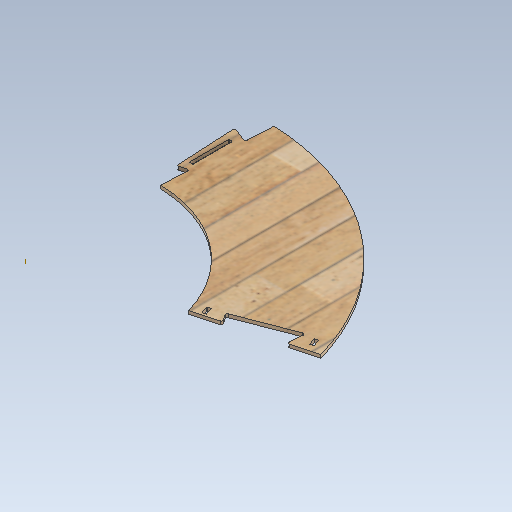
# Autodesk Inventor part: Ring C3
Saved by Autodesk Inventor 2020 (Build 240168000, 168)
## iProperties
Created: 2020-03-10
Part Number: Ring C3
Material: Wood (Maple)
Document SubType Name: Sheet Metal
Designer: Daniel Wikman
Density: 0.67 g/cm^3
Sheet Metal Rule: Default_mm
Appearance: Natural Maple - Glossy Dark Tint
Author: Daniel Wikman
Autodesk Inventor part; units mm, degrees
ref_plane "YZ Plane" through (0, 0, 0) normal (1, 0, 0) x (0, 1, 0)
ref_plane "XZ Plane" through (0, 0, 0) normal (0, 1, 0) x (-1, 0, 0)
ref_plane "XY Plane" through (0, 0, 0) normal (0, 0, 1) x (1, 0, 0)
sketch "Sketch1" plane through (0, 0, 0) normal (0, 1, 0) x (-1, 0, 0)
  circle A0 centre (0, 0) radius 425
  circle A1 centre (0, 0) radius 233.71
  dimension "d84" = 467.42
  dimension "d85" = 850
  constraints: 2 centre point, 1 coincident
  measures "d84" diameter of A1
  measures "d85" diameter of A0
extrude "Extrusion3" add sketch "Sketch1" along normal blind 6
sketch "Sketch2" plane through (0, 6, 0) normal (0, 1, 0) x (1, 0, 0)
  circle A0 centre (0, 0) radius 329.355 construction
  line L0 (3.25, 363.0217) -> (3.25, 295.6883)
  line L1 (-3.25, 295.6883) -> (-3.25, 363.0217)
  arc A1 (-3.25, 295.6883) -> (-1.9167, 294.355) centre (-1.9167, 295.6883) ccw
  arc A2 (1.9167, 294.355) -> (3.25, 295.6883) centre (1.9167, 295.6883) ccw
  arc A3 (-1.9167, 364.355) -> (-3.25, 363.0217) centre (-1.9167, 363.0217) ccw
  arc A4 (3.25, 363.0217) -> (1.9167, 364.355) centre (1.9167, 363.0217) ccw
  line L2 (-1.9167, 364.355) -> (1.9167, 364.355)
  line L3 (-1.9167, 294.355) -> (1.9167, 294.355)
  line L4 (0, 294.355) -> (0, 329.355) construction
  line L5 (0, 364.355) -> (0, 329.355) construction
  line L6 (0, 364.355) -> (0, 294.355) construction
  line L7 (175.0629, -238.5433) -> (171.9617, -240.7965)
  arc A5 (176.9253, -238.8383) -> (175.0629, -238.5433) centre (175.8467, -239.622) ccw
  arc A6 (171.9617, -240.7965) -> (171.6667, -242.6589) centre (172.7454, -241.8752) ccw
  line L8 (173.0175, -238.1382) -> (193.59, -266.4538) construction
  line L9 (211.2443, -297.1327) -> (171.6667, -242.6589)
  line L10 (176.9253, -238.8383) -> (216.5029, -293.3121)
  line L11 (214.1625, -294.7694) -> (173.0175, -238.1382) construction
  line L12 (214.1625, -294.7694) -> (193.59, -266.4538) construction
  arc A7 (211.2443, -297.1327) -> (213.1067, -297.4277) centre (212.323, -296.349) ccw
  line L13 (216.2079, -295.1745) -> (213.1067, -297.4277)
  arc A8 (216.2079, -295.1745) -> (216.5029, -293.3121) centre (215.4242, -294.0958) ccw
  line L14 (280.1548, 92.2019) -> (281.3393, 88.5562)
  arc A9 (281.0108, 93.882) -> (280.1548, 92.2019) centre (281.4229, 92.614) ccw
  arc A10 (281.3393, 88.5562) -> (283.0194, 87.7002) centre (282.6074, 88.9682) ccw
  line L15 (279.9482, 90.9607) -> (313.2352, 101.7763) construction
  line L16 (347.0573, 108.5073) -> (283.0194, 87.7002)
  line L17 (281.0108, 93.882) -> (345.0486, 114.6892)
  line L18 (346.5222, 112.5919) -> (279.9482, 90.9607) construction
  line L19 (346.5222, 112.5919) -> (313.2352, 101.7763) construction
  arc A11 (347.0573, 108.5073) -> (347.9133, 110.1874) centre (346.6452, 109.7754) ccw
  line L20 (346.7287, 113.8331) -> (347.9133, 110.1874)
  arc A12 (346.7287, 113.8331) -> (345.0486, 114.6892) centre (345.4607, 113.4211) ccw
  dimension "d86" = 658.71
  dimension "d21" = 6.5
  dimension "d24" = 2.6667
  dimension "d25" = 2.6667
  dimension "d32" = 1.3333
  dimension "d33" = 1.3333
  dimension "d162" = 70
  dimension "d163" = 294.355
  dimension "d165" = 3.25
  constraints: 42 end point, 24 point on circle, 12 centre point, 8 tangent, 2 midpoint, 1 coincident, 1 parallel, 1 vertical, 1 vertical alignment, 3 other
  measures "d21" distance between parallel lines of L0 L1
  measures "d24" diameter of A1
  measures "d25" diameter of A2
  measures "d32" radius of A3
  measures "d33" radius of A4
  measures "d162" distance between parallel lines of L3 L2
  measures "d163" distance from line of point (0, 0) L3
  measures "d165" distance between parallel lines of L5 L1
extrude "Extrusion4" cut sketch "Sketch2" against normal through all
sketch "Sketch3" plane through (0, 6, 0) normal (0, 1, 0) x (1, 0, 0)
  arc A0 (-131.3389, -404.1968) -> (131.3445, -404.195) centre (0, 0) ccw
  arc A1 (-77.7244, -128.3741) -> (77.7297, -128.3709) centre (0, 0) ccw
  line L0 (-122.1811, -173.696) -> (-161.3589, -227.6196)
  line L1 (-131.3389, -404.1968) -> (-77.7244, -128.3741)
  line L2 (0, 0) -> (0, -341.2918)
  line L3 (131.3445, -404.195) -> (77.7297, -128.3709)
  line L4 (210.5535, -295.3313) -> (171.3679, -241.3969) projected
  dimension "d52" = 25
  dimension "d87" = 150.07
  dimension "d88" = 425
  dimension "d89" = 25
  dimension "d90" = 11
  dimension "d91" = 11
  constraints: 8 end point, 4 point on circle, 2 centre point, 1 coincident
  measures "d52" angle of L0 L1
  measures "d87" radius of A1
  measures "d88" radius of A0
  measures "d89" angle of L4 L3
  measures "d90" angle of L3 L2
  measures "d91" angle of L1 L2
sketch "Sketch5" plane through (0, 6, 0) normal (0, 1, 0) x (1, 0, 0)
  line L0 (3.25, 363.0217) -> (3.25, 295.6883) projected
  line L1 (5.5862, 281.6788) -> (-6.155, 278.5328)
  line L2 (-11.2263, 385.43) -> (10.5847, 377.0575)
  line L3 (6.5657, 233.6709) -> (8.9394, 278.9635)
  line L4 (14.2034, 379.4075) -> (16.5771, 424.7001)
  arc A0 (10.5847, 377.0575) -> (14.2034, 379.4075) centre (11.5404, 379.5471) ccw
  arc A1 (8.9394, 278.9635) -> (5.5862, 281.6788) centre (6.2763, 279.103) ccw
  arc A2 (-11.2263, 385.43) -> (-14.8449, 382.8009) centre (-12.1819, 382.9405) ccw
  line L5 (-3.25, 295.6883) -> (-3.25, 363.0217) projected
  line L6 (-14.8449, 382.8009) -> (-9.5081, 280.969)
  arc A3 (-9.5081, 280.969) -> (-6.155, 278.5328) centre (-6.8451, 281.1086) ccw
  line L7 (-1.9167, 294.355) -> (1.9167, 294.355) projected
  line L8 (1.9167, 364.355) -> (-1.9167, 364.355) projected
  line L9 (16.5771, 424.7001) -> (16.5774, 424.7058)
  line L10 (6.5657, 233.6709) -> (6.5621, 233.6028)
  circle A4 centre (0, 0) radius 425
  circle A5 centre (0, 0) radius 233.71
  line L11 (-356.4489, 130.7516) -> (-398.7912, 147.0053)
  arc A6 (-355.3322, 126.5839) -> (-356.4489, 130.7516) centre (-357.4046, 128.2621) ccw
  line L12 (-370.0348, 108.4276) -> (-355.3322, 126.5839)
  arc A7 (-370.0348, 108.4276) -> (-368.6526, 104.1736) centre (-367.9624, 106.7494) ccw
  line L13 (-368.6526, 104.1736) -> (-270.1556, 77.7814)
  arc A8 (-270.1556, 77.7814) -> (-266.8024, 80.2177) centre (-269.4654, 80.3572) ccw
  line L14 (-266.1663, 92.3563) -> (-266.8024, 80.2177)
  arc A9 (-262.5476, 94.7063) -> (-266.1663, 92.3563) centre (-263.5032, 92.2167) ccw
  line L15 (-220.2053, 78.4526) -> (-262.5476, 94.7063)
  line L16 (-220.2053, 78.4526) -> (-220.1417, 78.4282)
  line L17 (-398.7912, 147.0053) -> (-398.7965, 147.0073)
  line L18 (-142.66, -185.1845) -> (-142.6172, -185.1316)
  line L19 (-263.0436, -333.8458) -> (-263.0472, -333.8502)
  line L20 (132.0366, -192.9029) -> (131.9995, -192.8458)
  line L21 (236.2213, -353.3334) -> (236.2244, -353.3381)
  line L22 (365.2271, 103.7351) -> (409.0364, 115.4738)
  arc A10 (361.8739, 106.4505) -> (365.2271, 103.7351) centre (364.5369, 106.3109) ccw
  line L23 (363.0966, 129.7812) -> (361.8739, 106.4505)
  arc A11 (363.0966, 129.7812) -> (359.478, 132.4103) centre (360.4336, 129.9208) ccw
  line L24 (359.478, 132.4103) -> (264.2793, 95.867)
  arc A12 (264.2793, 95.867) -> (262.9985, 91.9251) centre (265.2349, 93.3774) ccw
  line L25 (269.6187, 81.7308) -> (262.9985, 91.9251)
  arc A13 (268.0724, 77.7026) -> (269.6187, 81.7308) centre (267.3822, 80.2784) ccw
  line L26 (224.2631, 65.9639) -> (268.0724, 77.7026)
  line L27 (224.2631, 65.9639) -> (224.1973, 65.9463)
  line L28 (409.0364, 115.4738) -> (409.0419, 115.4753)
  line L29 (0, -233.71) -> (0, -425)
  arc A14 (131.3445, -404.195) -> (-131.3389, -404.1968) centre (0, 0) ccw projected
  point P0 (-425, 0)
  point P1 (-425, 0)
  point P2 (-398.7693, 146.9969)
  point P3 (-220.1557, 78.4336)
  point P4 (16.5759, 424.6766)
  point P5 (6.5629, 233.6178)
  point P6 (409.0137, 115.4677)
  point P7 (224.2118, 65.9502)
  dimension "d63" = 2.6667
  dimension "d64" = 3
  dimension "d66" = 3
  dimension "d67" = 2.6667
  dimension "d68" = 2.6667
  dimension "d70" = 72
  dimension "d71" = 72
  constraints: 52 end point, 26 point on circle, 13 centre point, 8 tangent, 2 collinear, 1 coincident, 1 equal radius, 1 vertical, 3 other
  measures "d63" radius of A0
  measures "d64" angle of L0 L4
  measures "d66" angle of L5 L6
  measures "d67" radius of A2
  measures "d68" radius of A3
  measures "d70" angle of L3 L1
  measures "d71" angle of L4 L2
sketch "Sketch6" plane through (0, 6, 0) normal (0, 1, 0) x (1, 0, 0)
  line L0 (237.9351, -331.8846) -> (247.6433, -324.8312)
  line L1 (243.8227, -319.5725) -> (234.1145, -326.626)
  line L2 (210.5535, -295.3313) -> (171.3679, -241.3969) projected
  line L3 (215.5172, -293.3731) -> (212.416, -295.6263) projected
  arc A0 (244.7539, -319.72) -> (243.8227, -319.5725) centre (244.2145, -320.1119) ccw
  arc A1 (247.6433, -324.8312) -> (247.7908, -323.9) centre (247.2514, -324.2918) ccw
  arc A2 (237.0039, -331.7371) -> (237.9351, -331.8846) centre (237.5432, -331.3452) ccw
  arc A3 (234.1145, -326.626) -> (233.967, -327.5572) centre (234.5063, -327.1653) ccw
  line L4 (233.967, -327.5572) -> (237.0039, -331.7371)
  line L5 (247.7908, -323.9) -> (244.7539, -319.72)
  line L6 (171.3679, -241.3969) -> (210.5535, -295.3313) projected
  line L7 (190.9607, -268.3641) -> (196.2193, -264.5435)
  line L8 (215.8122, -291.5107) -> (176.6265, -237.5763) projected
  line L9 (145.065, -204.0599) -> (154.7732, -197.0065)
  line L10 (158.5938, -202.2651) -> (148.8856, -209.3185)
  arc A4 (158.5938, -202.2651) -> (158.7413, -201.3339) centre (158.202, -201.7257) ccw
  arc A5 (155.7044, -197.154) -> (154.7732, -197.0065) centre (155.1651, -197.5458) ccw
  arc A6 (145.065, -204.0599) -> (144.9175, -204.9911) centre (145.4569, -204.5992) ccw
  arc A7 (147.9544, -209.171) -> (148.8856, -209.3185) centre (148.4938, -208.7792) ccw
  line L11 (147.9544, -209.171) -> (144.9175, -204.9911)
  line L12 (155.7044, -197.154) -> (158.7413, -201.3339)
  point P0 (0, 0)
  dimension "d104" = 6.5
  dimension "d105" = 12
  dimension "d108" = 1.3333
  dimension "d109" = 1.3333
  dimension "d110" = 1.3333
  dimension "d111" = 1.3333
  dimension "d112" = 0
  dimension "d149" = 145
  dimension "d150" = 90
  dimension "d151" = 90
  dimension "d152" = 90
  dimension "d153" = 90
  constraints: 18 end point, 16 point on circle, 12 symmetric about line, 8 centre point, 8 tangent, 2 midpoint, 4 other
  measures "d104" distance of L1.end L0.start
  measures "d105" distance of L0.start L0.end
  measures "d108" diameter of A0
  measures "d109" diameter of A1
  measures "d110" diameter of A2
  measures "d111" diameter of A3
  measures "d112" distance between parallel lines of L2 L4
  measures "d149" diameter of L1 L7
  measures "d150" angle of L5 L1
  measures "d151" angle of L0 L5
  measures "d152" angle of L4 L0
  measures "d153" angle of L1 L4
extrude "Extrusion7" cut sketch "Sketch6" against normal through all
pattern_circular "Circular Pattern2" count 2 over 72 about axis through (0, -10, 0) along (0, 1, 0) of "Extrusion7"
pattern_circular "Circular Pattern3" count 2 over 144 about axis through (0, -10, 0) along (0, 1, 0) of "Extrusion7"
mirror "Mirror3" about plane through (0, 0, 0) normal (1, 0, 0) of "Extrusion7"
extrude "Extrusion10" cut sketch "Sketch3" against normal blind 10
mirror "Mirror4" about plane through (0, 0, 0) normal (1, 0, 0) of "Extrusion4"
pattern_circular "Circular Pattern4" count 2 over 144 about axis through (0, -10, 0) along (0, -1, 0) of "Extrusion7"
extrude "Extrusion11" cut sketch "Sketch5" against normal through all contours A1 L3 L10 A5 L16 L15 A9 L14 A8 L13 A7 L12 A6 L11 A4 L4 A0 L2 A2 L6 A3 L1 | L27 L26 A13 L25 A12 L24 A11 L23 A10 L22 A4 L29 A5 | A5 L29 A4 L11 A6 L12 A7 L13 A8 L14 A9 L15 L16
equation "\"BendRadius\" = Thickness"
equation "\"BendReliefWidth\" = Thickness"
equation "\"BendReliefDepth\" = 0.5 * Thickness"
equation "\"CornerReliefSize\" = 4 * Thickness"
equation "\"MinimumRemnant\" = 2 * Thickness"
equation "\"TransitionRadius\" = BendRadius"
equation "\"JacobiRadiusSize\" = BendRadius"
equation "\"GapSize\" = Thickness"
equation "\"Thickness\" = 0.5"
body "Solid3"
